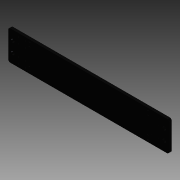
# Autodesk Inventor part: GANTRY CROSS PLATE
Saved by Autodesk Inventor 2013 (Build 170138000, 138)
## iProperties
Created: 2014-03-03
Part Number: GANTRY CROSS PLATE
Material: Generic
Document SubType Name: Modeling
Designer: employee
Density: 1 g/cm^3
Author: employee
Autodesk Inventor part; units mm, degrees
ref_plane "YZ Plane" through (0, 0, 0) normal (1, 0, 0) x (0, 1, 0)
ref_plane "XZ Plane" through (0, 0, 0) normal (0, 1, 0) x (-1, 0, 0)
ref_plane "XY Plane" through (0, 0, 0) normal (0, 0, 1) x (1, 0, 0)
sketch "Sketch1" plane through (0, 0, 0) normal (0, 0, 1) x (1, 0, 0)
  arc A0 (-299.7867, -35) -> (-294.7867, -30) centre (-299.7867, -30) ccw projected
  line L0 (-294.7867, -30) -> (-294.7867, 30) projected
  arc A1 (-294.7867, 30) -> (-299.7867, 35) centre (-299.7867, 30) ccw projected
  line L1 (-299.7867, 35) -> (-344.7867, 35) projected
  arc A2 (-344.7867, 35) -> (-349.7867, 30) centre (-344.7867, 30) ccw projected
  line L2 (-349.7867, 30) -> (-349.7867, -30) projected
  arc A3 (-349.7867, -30) -> (-344.7867, -35) centre (-344.7867, -30) ccw projected
  line L3 (-344.7867, -35) -> (-299.7867, -35) projected
  circle A4 centre (-338.7867, -12.5) radius 4 projected
  circle A5 centre (-338.7867, 12.5) radius 4 projected
  line L4 (-301.7867, -21) -> (-301.7867, -19.5) projected
  line L5 (-301.7867, -19.5) -> (-297.7867, -19.5) projected
  line L6 (-297.7867, -19.5) -> (-297.7867, -21) projected
  line L7 (-297.7867, -21) -> (-301.7867, -21) projected
  line L8 (-326.2867, -15.5) -> (-326.2867, -11.5) projected
  line L9 (-326.2867, -11.5) -> (-324.7867, -11.5) projected
  line L10 (-324.7867, -11.5) -> (-324.7867, -15.5) projected
  line L11 (-324.7867, -15.5) -> (-326.2867, -15.5) projected
  line L12 (-309.7867, -15.5) -> (-309.7867, -11.5) projected
  line L13 (-309.7867, -11.5) -> (-308.2867, -11.5) projected
  line L14 (-308.2867, -11.5) -> (-308.2867, -15.5) projected
  line L15 (-308.2867, -15.5) -> (-309.7867, -15.5) projected
  line L16 (-324.7867, -25.5) -> (-324.7867, -29.5) projected
  line L17 (-324.7867, -29.5) -> (-326.2867, -29.5) projected
  line L18 (-326.2867, -29.5) -> (-326.2867, -25.5) projected
  line L19 (-326.2867, -25.5) -> (-324.7867, -25.5) projected
  line L20 (-308.2867, -25.5) -> (-308.2867, -29.5) projected
  line L21 (-308.2867, -29.5) -> (-309.7867, -29.5) projected
  line L22 (-309.7867, -29.5) -> (-309.7867, -25.5) projected
  line L23 (-309.7867, -25.5) -> (-308.2867, -25.5) projected
  line L24 (-297.7867, -29) -> (-297.7867, -30.5) projected
  line L25 (-297.7867, -30.5) -> (-301.7867, -30.5) projected
  line L26 (-301.7867, -30.5) -> (-301.7867, -29) projected
  line L27 (-301.7867, -29) -> (-297.7867, -29) projected
  line L28 (-309.7867, 29.5) -> (-308.2867, 29.5) projected
  line L29 (-308.2867, 29.5) -> (-308.2867, 25.5) projected
  line L30 (-308.2867, 25.5) -> (-309.7867, 25.5) projected
  line L31 (-309.7867, 25.5) -> (-309.7867, 29.5) projected
  line L32 (-326.2867, 25.5) -> (-326.2867, 29.5) projected
  line L33 (-326.2867, 29.5) -> (-324.7867, 29.5) projected
  line L34 (-324.7867, 29.5) -> (-324.7867, 25.5) projected
  line L35 (-324.7867, 25.5) -> (-326.2867, 25.5) projected
  line L36 (-308.2867, 11.5) -> (-309.7867, 11.5) projected
  line L37 (-309.7867, 11.5) -> (-309.7867, 15.5) projected
  line L38 (-309.7867, 15.5) -> (-308.2867, 15.5) projected
  line L39 (-308.2867, 15.5) -> (-308.2867, 11.5) projected
  line L40 (-324.7867, 15.5) -> (-324.7867, 11.5) projected
  line L41 (-324.7867, 11.5) -> (-326.2867, 11.5) projected
  line L42 (-326.2867, 11.5) -> (-326.2867, 15.5) projected
  line L43 (-326.2867, 15.5) -> (-324.7867, 15.5) projected
  line L44 (-297.7867, 19.5) -> (-301.7867, 19.5) projected
  line L45 (-301.7867, 19.5) -> (-301.7867, 21) projected
  line L46 (-301.7867, 21) -> (-297.7867, 21) projected
  line L47 (-297.7867, 21) -> (-297.7867, 19.5) projected
  line L48 (-301.7867, 29) -> (-301.7867, 30.5) projected
  line L49 (-301.7867, 30.5) -> (-297.7867, 30.5) projected
  line L50 (-297.7867, 30.5) -> (-297.7867, 29) projected
  line L51 (-297.7867, 29) -> (-301.7867, 29) projected
  arc A6 (-19.7867, 35) -> (-24.7867, 30) centre (-19.7867, 30) ccw projected
  line L52 (-24.7867, 30) -> (-24.7867, -30) projected
  arc A7 (-24.7867, -30) -> (-19.7867, -35) centre (-19.7867, -30) ccw projected
  line L53 (-19.7867, -35) -> (25.2133, -35) projected
  arc A8 (25.2133, -35) -> (30.2133, -30) centre (25.2133, -30) ccw projected
  line L54 (30.2133, -30) -> (30.2133, 30) projected
  arc A9 (30.2133, 30) -> (25.2133, 35) centre (25.2133, 30) ccw projected
  line L55 (25.2133, 35) -> (-19.7867, 35) projected
  circle A10 centre (19.2133, 12.5) radius 4 projected
  circle A11 centre (19.2133, -12.5) radius 4 projected
  line L56 (-17.7867, 21) -> (-17.7867, 19.5) projected
  line L57 (-17.7867, 19.5) -> (-21.7867, 19.5) projected
  line L58 (-21.7867, 19.5) -> (-21.7867, 21) projected
  line L59 (-21.7867, 21) -> (-17.7867, 21) projected
  line L60 (6.7133, 15.5) -> (6.7133, 11.5) projected
  line L61 (6.7133, 11.5) -> (5.2133, 11.5) projected
  line L62 (5.2133, 11.5) -> (5.2133, 15.5) projected
  line L63 (5.2133, 15.5) -> (6.7133, 15.5) projected
  line L64 (-9.7867, 15.5) -> (-9.7867, 11.5) projected
  line L65 (-9.7867, 11.5) -> (-11.2867, 11.5) projected
  line L66 (-11.2867, 11.5) -> (-11.2867, 15.5) projected
  line L67 (-11.2867, 15.5) -> (-9.7867, 15.5) projected
  line L68 (5.2133, 25.5) -> (5.2133, 29.5) projected
  line L69 (5.2133, 29.5) -> (6.7133, 29.5) projected
  line L70 (6.7133, 29.5) -> (6.7133, 25.5) projected
  line L71 (6.7133, 25.5) -> (5.2133, 25.5) projected
  line L72 (-11.2867, 25.5) -> (-11.2867, 29.5) projected
  line L73 (-11.2867, 29.5) -> (-9.7867, 29.5) projected
  line L74 (-9.7867, 29.5) -> (-9.7867, 25.5) projected
  line L75 (-9.7867, 25.5) -> (-11.2867, 25.5) projected
  line L76 (-21.7867, 29) -> (-21.7867, 30.5) projected
  line L77 (-21.7867, 30.5) -> (-17.7867, 30.5) projected
  line L78 (-17.7867, 30.5) -> (-17.7867, 29) projected
  line L79 (-17.7867, 29) -> (-21.7867, 29) projected
  line L80 (-9.7867, -29.5) -> (-11.2867, -29.5) projected
  line L81 (-11.2867, -29.5) -> (-11.2867, -25.5) projected
  line L82 (-11.2867, -25.5) -> (-9.7867, -25.5) projected
  line L83 (-9.7867, -25.5) -> (-9.7867, -29.5) projected
  line L84 (6.7133, -25.5) -> (6.7133, -29.5) projected
  line L85 (6.7133, -29.5) -> (5.2133, -29.5) projected
  line L86 (5.2133, -29.5) -> (5.2133, -25.5) projected
  line L87 (5.2133, -25.5) -> (6.7133, -25.5) projected
  line L88 (-11.2867, -11.5) -> (-9.7867, -11.5) projected
  line L89 (-9.7867, -11.5) -> (-9.7867, -15.5) projected
  line L90 (-9.7867, -15.5) -> (-11.2867, -15.5) projected
  line L91 (-11.2867, -15.5) -> (-11.2867, -11.5) projected
  line L92 (5.2133, -15.5) -> (5.2133, -11.5) projected
  line L93 (5.2133, -11.5) -> (6.7133, -11.5) projected
  line L94 (6.7133, -11.5) -> (6.7133, -15.5) projected
  line L95 (6.7133, -15.5) -> (5.2133, -15.5) projected
  line L96 (-21.7867, -19.5) -> (-17.7867, -19.5) projected
  line L97 (-17.7867, -19.5) -> (-17.7867, -21) projected
  line L98 (-17.7867, -21) -> (-21.7867, -21) projected
  line L99 (-21.7867, -21) -> (-21.7867, -19.5) projected
  line L100 (-17.7867, -29) -> (-17.7867, -30.5) projected
  line L101 (-17.7867, -30.5) -> (-21.7867, -30.5) projected
  line L102 (-21.7867, -30.5) -> (-21.7867, -29) projected
  line L103 (-21.7867, -29) -> (-17.7867, -29) projected
  line L104 (-299.7867, 35) -> (-19.7867, 35)
  line L105 (-19.7867, -35) -> (-299.7867, -35)
  point P0 (0, 0)
  constraints: 4 end point, 4 tangent, 1 collinear, 1 parallel
extrude "Extrusion1" add sketch "Sketch1" along normal blind 6.477
body "Solid1"
